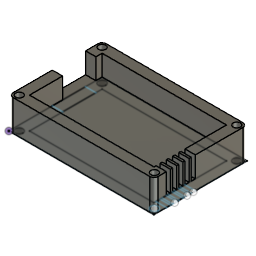
Case for esp32 (Autodesk Fusion 360 design; units mm, degrees)
part number: 2025-12-27-14-16-15-248
Autodesk Fusion 360 part; units mm, degrees
sketch "Sketch1" plane through (0, 0, 0) normal (0, 0, 1) x (1, 0, 0)
  line L0 (0, 0) -> (70, 0)
  line L1 (70, 0) -> (70, 45)
  line L2 (70, 45) -> (0, 45)
  line L3 (0, 45) -> (0, 0)
  line L4 (5, 40) -> (65, 40)
  line L5 (65, 40) -> (65, 5)
  line L6 (65, 5) -> (5, 5)
  line L7 (5, 5) -> (5, 40)
  line L8 (70, 19) -> (70, 21)
  line L9 (70, 16) -> (70, 18)
  line L10 (65, 18) -> (65, 16)
  line L11 (65, 15) -> (65, 13)
  line L12 (70, 10) -> (70, 12)
  line L13 (65, 12) -> (65, 10)
  line L14 (0, 37) -> (5, 37)
  line L15 (5, 37) -> (5, 21)
  line L16 (5, 21) -> (0, 21)
  line L17 (0, 21) -> (0, 37)
  line L18 (65, 18) -> (70, 18)
  line L19 (70, 18) -> (70, 20)
  line L20 (70, 20) -> (65, 20)
  line L21 (65, 20) -> (65, 18)
  line L22 (65, 15) -> (70, 15)
  line L23 (70, 15) -> (70, 17)
  line L24 (70, 17) -> (65, 17)
  line L25 (65, 17) -> (65, 15)
  line L26 (65, 12) -> (70, 12)
  line L27 (70, 12) -> (70, 14)
  line L28 (70, 14) -> (65, 14)
  line L29 (65, 14) -> (65, 12)
  line L30 (65, 11) -> (70, 11)
  line L31 (70, 11) -> (70, 9)
  line L32 (70, 9) -> (65, 9)
  line L33 (65, 9) -> (65, 11)
  line L34 (70, 8) -> (65, 8)
  line L35 (65, 8) -> (65, 6)
  line L36 (65, 6) -> (70, 6)
  line L37 (70, 6) -> (70, 8)
  circle A0 centre (67.5, 42.5) radius 1.75
  circle A1 centre (2.5, 2.5) radius 1.75
  circle A2 centre (2.5, 42.5) radius 1.75
  circle A3 centre (67.5, 2.7406) radius 1.75
  point P0 (-50.3404, 3.4837)
  dimension "d1" = 45
  dimension "d2" = 70
  dimension "d3" = 35
  dimension "d4" = 60
  dimension "d5" = 5
  dimension "d6" = 5
  dimension "d7" = 16
  dimension "d8" = 3.5
  dimension "d9" = 2.5
  dimension "d10" = 2.5
  dimension "d11" = 3.5
  dimension "d12" = 2.5
  dimension "d13" = 2.5
  dimension "d14" = 3.5
  dimension "d15" = 2.5
  dimension "d16" = 2.5
  dimension "d17" = 3.5
  dimension "d18" = 2.5
  constraint horizontal L0
  constraint vertical L1
  constraint horizontal L2
  constraint vertical L3
  constraint coincident L0.start L3.end
  constraint horizontal L4
  constraint vertical L5
  constraint horizontal L6
  constraint vertical L7
  constraint vertical L8
  constraint coincident L1 L8.end
  constraint vertical L9
  constraint vertical L10
  constraint coincident L1 L9.end
  constraint coincident L5 L10.end
  constraint vertical L11
  constraint coincident L5 L11.end
  constraint vertical L12
  constraint vertical L13
  constraint coincident L1 L12.end
  constraint coincident L5 L13.end
  constraint horizontal L14
  constraint vertical L15
  constraint horizontal L16
  constraint vertical L17
  constraint coincident L7 L15.end
  constraint coincident L3 L14.start
  constraint horizontal L18
  constraint vertical L19
  constraint horizontal L20
  constraint vertical L21
  constraint midpoint L8 L19.end
  constraint horizontal L22
  constraint vertical L23
  constraint horizontal L24
  constraint vertical L25
  constraint midpoint L9 L23.end
  constraint horizontal L26
  constraint vertical L27
  constraint horizontal L28
  constraint vertical L29
  constraint coincident L1 L27.end
  constraint horizontal L30
  constraint vertical L31
  constraint horizontal L32
  constraint vertical L33
  constraint midpoint L13 L30.start
  constraint horizontal L34
  constraint vertical L35
  constraint horizontal L36
  constraint vertical L37
  constraint coincident L5 L35.end
  constraint coincident L1 L34.start
  measures "d1" distance of L0.start L2.end
  measures "d2" distance of L1.end L2.end
  measures "d3" distance of L4.start L6.end
  measures "d4" distance of L4.start L4.end
  measures "d5" horizontal distance of L1.end L4.end
  measures "d6" vertical distance of L0.start L6.end
  measures "d7" distance of L14.start L16.end
  measures "d8" diameter of A0
  measures "d9" vertical distance of L1.end A0.centre
  measures "d10" horizontal distance of L1.end A0.centre
  measures "d11" diameter of A1
  measures "d12" horizontal distance of L0.start A1.centre
  measures "d13" vertical distance of L0.start A1.centre
  measures "d14" diameter of A2
  measures "d15" vertical distance of L2.end A2.centre
  measures "d16" distance of L3 A2.centre
  measures "d17" diameter of A3
  measures "d18" horizontal distance of L0.end A3.centre
extrude "Extrude1" add sketch "Sketch1" along normal blind 15 contours L0 L1 L3 L5 L6 L7 L16 L36 | L1 L2 L3 L4 L5 L7 L8 L14 L20 | L1 L5 L32 L34 | L1 L5 L12 L13 L26 L30 | L1 L5 L9 L10 L18 L24 | L1 L5 L11 L22 L28 makes body 1 at (66.6667, 11, 5) makes body 2 at (46.6667, 45, 10) makes body 3 at (68.3333, 14, 5) makes body 4 at (68.3333, 9, 5) makes body 5 at (23.3333, 0, 10) makes body 6 at (66.6667, 18, 5)
extrude "Extrude2" add sketch "Sketch1" along normal blind 5 separate body contours L4 L5 L6 L7 L10 L11 L13 L15 L21 L25 L29 L33 L35 makes body 7
fillet "Fillet1" radius 2 4 edges at (70, 45, 7.5) (0, 45, 7.5) (70, 0, 7.5) (0, 0, 7.5) on bodies 2 5
extrude "Extrude3" add sketch "Sketch1" along normal blind 5 contours L3 L7 L14 L15 L16 L17 bodies 2 5 7
extrude "Extrude4" add sketch "Sketch1" along normal blind 5 contours L1 L5 L34 L35 L36 L37 | L1 L5 L12 L13 L30 L31 L32 L33 | L1 L5 L8 L18 L19 L20 L21 | L1 L5 L11 L26 L27 L28 L29 | L1 L5 L9 L10 L22 L23 L24 L25 bodies 1 2 3 4 6
